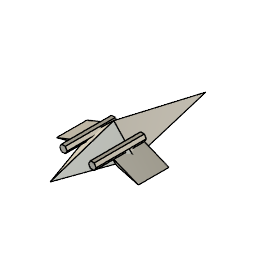
Typhoon (Autodesk Fusion 360 design; units mm, degrees)
Autodesk Fusion 360 part; units mm, degrees
sketch "Sketch1" plane through (0, 0, 0) normal (0, 0, 1) x (1, 0, 0)
  line L0 (0, 0) -> (0, 14000)
  line L1 (0, 0) -> (0, -14000)
  line L2 (0, 14000) -> (4000, -2780.7192)
  line L3 (4000, -2780.7192) -> (0, -14000)
  line L4 (0, 14000) -> (-4000, -2780.7192)
  line L5 (-4000, -2780.7192) -> (0, -14000)
  line L6 (-4000, -2780.7192) -> (4000, -2780.7192)
  dimension "d1" = 14000
  dimension "d2" = 14000
  constraint coincident L0.start L1.start
  constraint vertical L0
  constraint parallel L0 L1
  constraint symmetric L2.start L0 L4.start
  constraint symmetric L0 L1.end L3.end
  constraint symmetric L0 L2.end L4.end
  measures "d1" distance of L0.start L0.end
  measures "d2" distance of L0.start L1.end
extrude "Extrude1" add sketch "Sketch1" along normal blind 4000 draft -45 makes body 1
sketch "Sketch2" plane through (0, 0, 0) normal (0, 1, 0) x (1, 0, 0)
  line L0 (-4000, 0) -> (0, -3840.6297)
  line L1 (0, 0) -> (0, -3840.6297)
  line L2 (0, 0) -> (-4000, 0)
  line L3 (-3281.4615, -1355.195) -> (-2930.1788, -1935.6168)
  line L4 (-2930.1788, -1935.6168) -> (-2251.8774, -1921.608)
  line L5 (-2251.8774, -1921.608) -> (-1924.8587, -1327.1773)
  line L6 (-1924.8587, -1327.1773) -> (-2276.1414, -746.7555)
  line L7 (-2276.1414, -746.7555) -> (-2954.4428, -760.7643)
  line L8 (-2954.4428, -760.7643) -> (-3281.4615, -1355.195)
  line L9 (1924.8587, -1327.1773) -> (2276.1414, -746.7555)
  line L10 (2276.1414, -746.7555) -> (2954.4428, -760.7643)
  line L11 (2954.4428, -760.7643) -> (3281.4615, -1355.195)
  line L12 (3281.4615, -1355.195) -> (2930.1788, -1935.6168)
  line L13 (2251.8774, -1921.608) -> (1924.8587, -1327.1773)
  line L14 (2930.1788, -1935.6168) -> (2251.8774, -1921.608)
  point P0 (-2603.1601, -1341.1861)
  constraint coincident L0 P0
  constraint symmetric L1 L3.start L11.end
  constraint symmetric L1 L3.end L12.end
  constraint symmetric L1 L4.end L13.start
  constraint symmetric L1 L5.end L9.start
  constraint symmetric L1 L6.end L9.end
  constraint symmetric L1 L7.end L10.end
extrude "Extrude2" add sketch "Sketch2" against normal blind 9000 separate body contours L0 L5 L6 L7 L8 | L0 L3 L4 L5 L8 | L9 L10 L11 L12 L13 L14 makes body 2 at (3063.4491, -3000, 958.9079) makes body 3 at (-3063.4491, -3000, 958.9079)
sketch "Sketch3" plane through (0, 0, 0) normal (0, 1, 0) x (1, 0, 0)
  line L0 (0, 0) -> (0, -3840.6297)
  line L1 (0, -3840.6297) -> (4000, 0)
  line L2 (4000, 0) -> (0, 0)
  line L3 (-4000, 0) -> (0, -3840.6297)
  line L4 (0, -3840.6297) -> (0, 0)
  line L5 (0, 0) -> (-4000, 0)
  line L6 (2930.1788, -1935.6168) -> (3281.4615, -1355.195)
  line L7 (3281.4615, -1355.195) -> (2954.4428, -760.7643)
  line L8 (2954.4428, -760.7643) -> (2276.1414, -746.7555)
  line L9 (2276.1414, -746.7555) -> (1924.8587, -1327.1773)
  line L10 (1924.8587, -1327.1773) -> (2251.8774, -1921.608)
  line L11 (2251.8774, -1921.608) -> (2930.1788, -1935.6168)
  line L12 (-2954.4428, -760.7643) -> (-3281.4615, -1355.195)
  line L13 (-3281.4615, -1355.195) -> (-2930.1788, -1935.6168)
  line L14 (-2930.1788, -1935.6168) -> (-2251.8774, -1921.608)
  line L15 (-2251.8774, -1921.608) -> (-1924.8587, -1327.1773)
  line L16 (-1924.8587, -1327.1773) -> (-2276.1414, -746.7555)
  line L17 (-2276.1414, -746.7555) -> (-2954.4428, -760.7643)
  line L18 (4000, 0) -> (7863.7033, 1035.2762)
  line L19 (4000, 0) -> (8000, 0) construction
  line L20 (7863.7033, 1035.2762) -> (3041.9681, -919.8614)
  line L21 (0, 0) -> (0, -3840.6297)
  line L22 (-7863.7033, 1035.2762) -> (-3041.9681, -919.8614)
  line L23 (-4000, 0) -> (-7863.7033, 1035.2762)
  dimension "d8" = 15
  dimension "d9" = 4000
  constraint horizontal L19
  constraint coincident L1.end L2.start
  constraint coincident L7 L20.end
  constraint coincident L1 L20.end
  constraint symmetric L1.end L21 L3.start
  constraint symmetric L18.end L21 L22.start
  constraint symmetric L20.end L21 L22.end
  measures "d8" angle of L18 L19
  measures "d9" distance of L1.end L18.end
extrude "Extrude3" add sketch "Sketch3" against normal blind 5500 separate body contours L1 L18 L20 | L3 L22 L23 makes body 4 at (6256.4582, -1833.3333, -383.5637) makes body 5 at (-6256.4582, -1833.3333, -383.5637)
move_body "Move1" bodies 5 to x (1, 0, 0) y (0, 1, 0) z (0, 0, 1) at (500, 0, 0)
move_body "Move2" bodies 4 to x (1, 0, 0) y (0, 1, 0) z (0, 0, 1) at (-500, 0, 0)
